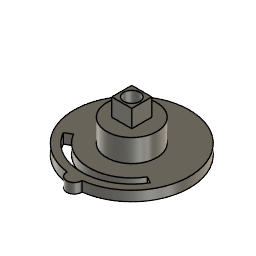
lens_selector (Autodesk Fusion 360 design; units mm, degrees)
Autodesk Fusion 360 part; units mm, degrees
note: some values were not read from the file. Set by a fixed rule: which sketch regions a step uses.
sketch "Sketch1" plane through (0, 0, 0) normal (0, 0, 1) x (1, 0, 0)
  circle A0 centre (0, -11.5) radius 2 construction
  circle A1 centre (0, 0) radius 12 construction
  circle A2 centre (0, -11.5) radius 1.5
  circle A3 centre (0, 0) radius 8.5
  line L0 (0, 0) -> (8.6603, -5)
  circle A4 centre (0, 0) radius 11.5
  line L1 (0, 0) -> (-8.6603, -5)
  circle A5 centre (0, 0) radius 10
  dimension "d4" = 1.5
  dimension "d5" = -1.5
  dimension "d6" = 2
  dimension "d7" = 0.5
  dimension "d8" = 20
  dimension "d9" = 3
  constraint coincident A1.centre A3.centre
  constraint coincident L0.end A5
  constraint coincident L1.end A5
  constraint coincident A0.centre A4
  measures "d8" diameter of A5
  measures "d9" diameter of A2
extrude "Extrude1" add sketch "Sketch1" along normal blind 2 contours A2 A4 | A2 A4 | A2 A4 | A3 L0 L1 A5 | A3 L0 L1 | A3 L0 L1 picked at (-8.9789, -3.0313)
sketch "Sketch2" plane through (0, 0, 2) normal (0, 0, 1) x (-1, 0, 0)
  arc A0 (7.3612, 4.25) -> (-7.3612, 4.25) centre (0, 0) ccw
  line L0 (-7.3612, 4.25) -> (-8.6603, 5)
  arc A1 (8.6603, 5) -> (-8.6603, 5) centre (0, 0) ccw
  line L1 (8.6603, 5) -> (7.3612, 4.25)
  arc A2 (-1.4968, 11.4022) -> (1.4968, 11.4022) centre (0, 0) ccw
  arc A3 (1.4968, 11.4022) -> (-1.4968, 11.4022) centre (0, 11.5) ccw
  circle A4 centre (0, 0) radius 5
  dimension "d12" = 10
  constraint concentric A0 A4
  measures "d12" diameter of A4
extrude "Extrude2" add sketch "Sketch2" along normal blind 4.5 contours A4
sketch "Sketch3" plane through (0, 0, 6.5) normal (0, 0, 1) x (-1, 0, 0)
  circle A0 centre (0, 0) radius 5
  line L0 (-2, 2) -> (2, 2)
  line L1 (2, 2) -> (2, -2)
  line L2 (2, -2) -> (-2, -2)
  line L3 (-2, -2) -> (-2, 2)
  constraint horizontal L0
  constraint vertical L1
  constraint horizontal L2
  constraint vertical L3
extrude "Extrude3" add sketch "Sketch3" along normal blind 3.5 contours L0 L1 L2 L3
sketch "Sketch4" plane through (0, 0, 0) normal (0, 0, -1) x (1, 0, 0)
  arc A0 (7.3612, 4.25) -> (-7.3612, 4.25) centre (0, 0) ccw
  line L0 (-7.3612, 4.25) -> (-8.6603, 5)
  arc A1 (8.6603, 5) -> (-8.6603, 5) centre (0, 0) ccw
  line L1 (8.6603, 5) -> (7.3612, 4.25)
  arc A2 (-1.4968, 11.4022) -> (1.4968, 11.4022) centre (0, 0) ccw
  arc A3 (1.4968, 11.4022) -> (-1.4968, 11.4022) centre (0, 11.5) ccw
  circle A4 centre (0, 0) radius 1.6
  line L2 (-1.5875, 2.7496) -> (-3.175, 0)
  line L3 (-3.175, 0) -> (-1.5875, -2.7496)
  line L4 (-1.5875, -2.7496) -> (1.5875, -2.7496)
  line L5 (1.5875, -2.7496) -> (3.175, 0)
  line L6 (3.175, 0) -> (1.5875, 2.7496)
  line L7 (1.5875, 2.7496) -> (-1.5875, 2.7496)
  dimension "d17" = 3.2
  dimension "d20" = 3.175
  constraint coincident A0.centre A1.centre
  measures "d17" diameter of A4
  measures "d20" distance of L2.start L6.end
extrude "Extrude4" cut sketch "Sketch4" against normal blind 3 contours L2 L3 L4 L5 L6 L7
extrude "Extrude5" cut 1 faces at (0.5286, -0.5507, 0) along direction (0, 0, 1) blind 10
